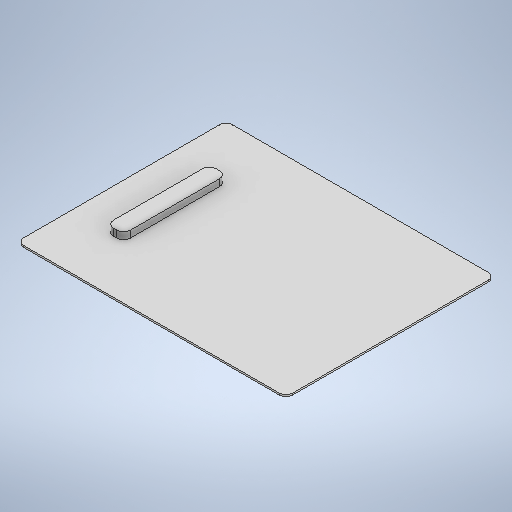
# Autodesk Inventor part: Tutup Pzem test1
Saved by Autodesk Inventor 2025.3 (Build 293356000, 356)
## iProperties
Created: 2026-02-07
Part Number: Tutup Pzem test1
Material: Generic
Document SubType Name: Modeling
Designer: Maulana
Density: 1 g/cm^3
Appearance: Default
Author: Maulana
Autodesk Inventor part; units mm, degrees
ref_plane "YZ Plane" through (0, 0, 0) normal (1, 0, 0) x (0, 1, 0)
ref_plane "XZ Plane" through (0, 0, 0) normal (0, 1, 0) x (-1, 0, 0)
ref_plane "XY Plane" through (0, 0, 0) normal (0, 0, 1) x (1, 0, 0)
sketch "Sketch3" plane through (0, 0, 0) normal (0, 1, 0) x (-1, 0, 0)
  line L0 (-39.25, 30.5) -> (39.25, 30.5)
  line L1 (39.25, 30.5) -> (39.25, -30.5)
  line L2 (39.25, -30.5) -> (-39.25, -30.5)
  line L3 (-39.25, -30.5) -> (-39.25, 30.5)
  line L4 (-39.25, 30.5) -> (39.25, -30.5) construction
  line L5 (39.25, 30.5) -> (-39.25, -30.5) construction
  point P0 (0, 0)
  dimension "d0" = 78.5
  dimension "d1" = 61
  constraints: 12 end point, 2 midpoint, 2 parallel, 1 horizontal, 1 perpendicular
  measures "d0" distance of L1.end L2.end
  measures "d1" distance of L0.end L1.end
extrude "Extrusion1" add sketch "Sketch3" along normal blind 0.5
sketch "Sketch4" plane through (0, 0.5, 0) normal (0, 1, 0) x (1, 0, 0)
  line L0 (-23.6083, -15) -> (-28.6083, -15)
  line L1 (-28.6083, -15) -> (-28.6083, 15)
  line L2 (-28.6083, 15) -> (-23.6083, 15)
  line L3 (-23.6083, 15) -> (-23.6083, -15)
  line L4 (-23.6083, -15) -> (-28.6083, 15) construction
  line L5 (-28.6083, -15) -> (-23.6083, 15) construction
  point P0 (0, 0)
  point P1 (-26.1083, 0)
  dimension "d4" = 5
  dimension "d5" = 30
  constraints: 12 end point, 2 midpoint, 2 parallel, 1 horizontal, 1 perpendicular
  measures "d4" distance of L1.end L2.end
  measures "d5" distance of L0.end L1.end
extrude "Extrusion2" add sketch "Sketch4" along normal blind 2
fillet "Fillet1" radius 2 4 edges at (-28.6083, 1.5, 15) (-23.6083, 1.5, 15) (-28.6083, 1.5, -15) (-23.6083, 1.5, -15)
fillet "Fillet2" radius 2 4 edges at (-39.25, 0.25, 30.5) (39.25, 0.25, 30.5) (39.25, 0.25, -30.5) (-39.25, 0.25, -30.5)
body "Solid1"
